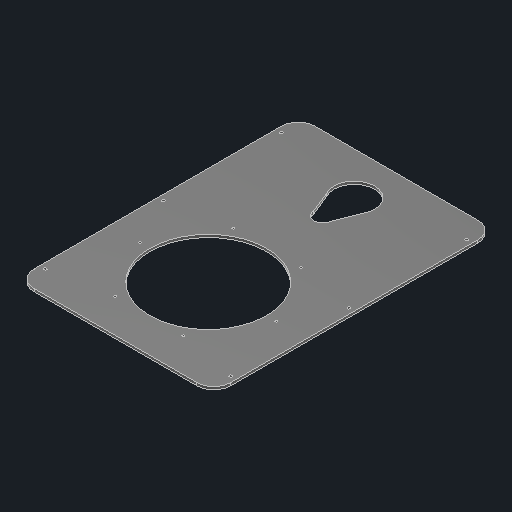
# Autodesk Inventor part: 부품8
Saved by Autodesk Inventor 2026.1 (Build 301233020, 233B)
## iProperties
Created: 2025-11-12
Part Number: 부품8
Material: ABS 플라스틱
Document SubType Name: Modeling
Designer: jaewook
Density: 1.06 g/cm^3
Appearance: 매끄러움 - 흰색
Author: jaewook
Autodesk Inventor part; units mm, degrees
ref_plane "YZ Plane" through (0, 0, 0) normal (1, 0, 0) x (0, 1, 0)
ref_plane "XZ Plane" through (0, 0, 0) normal (0, 1, 0) x (-1, 0, 0)
ref_plane "XY Plane" through (0, 0, 0) normal (0, 0, 1) x (1, 0, 0)
sketch "스케치1" plane through (0, 0, 0) normal (0, 1, 0) x (-1, 0, 0)
  line L0 (145, 250) -> (-145, 250)
  line L1 (-175, 220) -> (-175, -220)
  line L2 (-145, -250) -> (145, -250)
  line L3 (175, -220) -> (175, 220)
  line L4 (175, 250) -> (-175, -250) construction
  line L5 (-175, 250) -> (175, -250) construction
  circle A0 centre (0, -175) radius 36
  arc A1 (145, -250) -> (175, -220) centre (145, -220) ccw
  arc A2 (-175, -220) -> (-145, -250) centre (-145, -220) ccw
  arc A3 (-145, 250) -> (-175, 220) centre (-145, 220) ccw
  arc A4 (175, 220) -> (145, 250) centre (145, 220) ccw
  circle A5 centre (0, 85) radius 103.75
  point P0 (0, 0)
  dimension "d0" = 350
  dimension "d1" = 500
  dimension "d2" = 72
  dimension "d3" = 30
  dimension "d4" = 75
  dimension "d5" = 207.5
  dimension "d7" = 165
  constraints: 12 end point, 8 point on circle, 8 point on line, 8 tangent, 6 centre point, 3 equal radius, 2 midpoint, 2 parallel, 2 vertical alignment, 1 horizontal, 1 perpendicular
  measures "d0" distance of L5.end L4.end
  measures "d1" distance of L4.end L5.start
  measures "d2" diameter of A0
  measures "d3" radius of A1
  measures "d4" distance from line of A0.centre L2
  measures "d5" diameter of A5
  measures "d7" distance from line of L0 A5.centre
extrude "돌출1" add sketch "스케치1" along normal blind 5
sketch "스케치2" plane through (0, 0, 0) normal (0, -1, 0) x (1, 0, 0)
  line L0 (-145, 250) -> (145, 250) projected
  line L1 (-175, -220) -> (-175, 220) projected
  line L2 (145, -250) -> (-145, -250) projected
  line L3 (175, 220) -> (175, -220) projected
  circle A0 centre (165, 210) radius 2.5
  line L4 (0, 250) -> (0, -250) construction
  line L5 (-175, 0) -> (175, 0) construction
  circle A1 centre (165, -210) radius 2.5
  circle A2 centre (165, 0) radius 2.5
  circle A3 centre (-165, 210) radius 2.5
  circle A4 centre (-165, -210) radius 2.5
  circle A5 centre (-165, 0) radius 2.5
  point P0 (0, 0)
  dimension "d11" = 5
  dimension "d12" = 40
  dimension "d13" = 10
  dimension "d14" = 5
  dimension "d15" = 10
  constraints: 6 centre point, 4 end point, 4 midpoint, 4 symmetric about line, 1 point on line, 4 other
  measures "d11" diameter of A0
  measures "d12" distance from line of A0.centre L0
  measures "d13" distance from line of L3 A0.centre
  measures "d14" diameter of A2
  measures "d15" distance from line of L3 A2.centre
extrude "돌출2" cut sketch "스케치2" against normal through all
sketch "스케치3" plane through (0, 5, 0) normal (0, 1, 0) x (1, 0, 0)
  circle A0 centre (0, 175) radius 36 projected
  circle A1 centre (0, 175) radius 33.15
  line L0 (0, 175) -> (0, 119.3)
  circle A2 centre (-55.0502, 292.3468) radius 36
  line L1 (26.9254, 146.1085) -> (31.6003, 157.7541)
  line L2 (15.9944, 118.8781) -> (21.8404, 133.441)
  arc A3 (-15.9945, 118.88) -> (15.9944, 118.8781) centre (0, 119.3) ccw
  line L3 (-20.7535, 130.7351) -> (-15.9945, 118.88)
  line L4 (-31.5976, 157.7491) -> (-25.8385, 143.4026)
  circle A4 centre (-55.0502, 292.3468) radius 36
  circle A5 centre (-55.0502, 292.3468) radius 36
  line L5 (-20.7535, 130.7351) -> (-25.8385, 143.4026)
  line L6 (21.8404, 133.441) -> (26.9254, 146.1085)
  arc A6 (-13.9206, 113.7129) -> (13.92, 113.7112) centre (0, 119.3) ccw construction
  line L7 (13.92, 113.7112) -> (15.9944, 118.8781) construction
  line L8 (-13.9206, 113.7129) -> (-15.9945, 118.88) construction
  point P0 (0, 0)
  dimension "d18" = 12.7747
  dimension "d19" = 13.65
  dimension "d21" = 16
  dimension "d22" = 15
  dimension "d23" = 176.985
  dimension "d24" = 136.256
  dimension "d25" = 5.5678
  dimension "d26" = 5.5678
  dimension "d27" = 55.7
  dimension "d28" = 15.6925
  dimension "d29" = 13.65
  dimension "d31" = 43.744
  dimension "d32" = 43.744
  dimension "d33" = 43.744
  dimension "d34" = 12.5489
  dimension "d35" = 15.4593
  constraints: 18 end point, 6 centre point, 6 point on circle, 3 coincident, 2 collinear, 1 vertical, 5 other
  measures "d18" distance of L5.start L3.end
  measures "d19" distance of L5.start L5.end
  measures "d21" radius of A3
  measures "d22" radius of A6
  measures "d25" distance of L7.start L2.start
  measures "d26" distance of L8.start L3.end
  measures "d27" distance of L0.start L0.end
  measures "d28" distance of L2.start L6.start
  measures "d29" distance of L6.start L6.end
  measures "d31" angle of L2 L3
  measures "d32" angle of L6 L5
  measures "d33" angle of L1 L4
  measures "d34" distance of L6.end L1.end
  measures "d35" distance of L5.end L4.start
extrude "돌출3" cut sketch "스케치3" against normal blind 10 contours A0 L1 L6 L2 A3 L3 L5 L4
sketch "스케치4" plane through (0, 5, 0) normal (0, 1, 0) x (1, 0, 0)
  circle A0 centre (0, -85) radius 103.75 projected
  circle A1 centre (-0.0796, -85.0052) radius 104.02 projected
  line L0 (-0.0796, -85.0052) -> (-121.1411, -85.0052) construction
  line L1 (-0.0796, -85.0052) -> (120.9819, -85.0052) construction
  circle A2 centre (-121.1411, -85.0052) radius 1.8
  circle A3 centre (-60.566, -189.9139) radius 1.8
  circle A4 centre (60.5751, -189.9087) radius 1.8
  circle A5 centre (121.1411, -84.9948) radius 1.8
  circle A6 centre (60.566, 19.9139) radius 1.8
  circle A7 centre (-60.5751, 19.9087) radius 1.8
  point P0 (0, 0)
  dimension "d38" = 121.0615
  dimension "d39" = 180
  dimension "d40" = 3.6
  dimension "d43" = 360
  constraints: 6 centre point, 4 end point, 2 horizontal, 1 coincident, 1 collinear, 13 other
  measures "d38" distance of L0.start L0.end
  measures "d39" angle of L0 L1
  measures "d40" diameter of A2
extrude "돌출4" cut sketch "스케치4" against normal blind 10 contours A2 | A3 | A4 | A5 | A6 | A7
